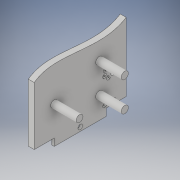
# Autodesk Inventor part: Case Right
Saved by Autodesk Inventor 2019 (Build 230136000, 136)
## iProperties
Created: 2022-04-25
Part Number: Case Right
Material: Generic
Document SubType Name: Modeling
Designer: Loxei
Density: 1 g/cm^3
Appearance: Default
Author: Loxei
Autodesk Inventor part; units mm, degrees
ref_plane "YZ Plane" through (0, 0, 0) normal (1, 0, 0) x (0, 1, 0)
ref_plane "XZ Plane" through (0, 0, 0) normal (0, 1, 0) x (-1, 0, 0)
ref_plane "XY Plane" through (0, 0, 0) normal (0, 0, 1) x (1, 0, 0)
sketch "Sketch1" plane through (0, 0, 0) normal (1, 0, 0) x (0, 1, 0)
  spline S0 degree 3 poles (-5.8666, 35) (13.8832, 21.2522) (-10.0462, -16.0043) (8.551, -35) knots 1 1 1 1 2 2 2 2
  line L0 (-5.8666, 35) -> (13.8832, 21.2522) construction
  line L1 (13.8832, 21.2522) -> (-10.0462, -16.0043) construction
  line L2 (-10.0462, -16.0043) -> (8.551, -35) construction
  line L3 (0, 65.172) -> (0, -65.172) construction
  line L4 (43.74, 0) -> (-43.74, 0) construction
  line L5 (-5.8666, 35) -> (-40.8666, 35)
  line L6 (-40.8666, 35) -> (-40.8666, 31)
  line L7 (-40.8666, 31) -> (-1.7165, 31)
  line L8 (-40.8666, 31) -> (-40.8666, -35)
  line L9 (-40.8666, -35) -> (8.551, -35)
  line L10 (-40.8666, -31) -> (5.392, -31)
  point P0 (0, 0)
  point P1 (0, 0)
  point P2 (-1.7165, 31)
  point P3 (0, 0)
  point P4 (0, 0)
  point P5 (0, 0)
  dimension "d0" = 35
  dimension "d1" = 4
  dimension "d2" = 4
  constraints: 16 end point, 4 midpoint, 3 perpendicular, 3 vertical, 2 horizontal, 2 parallel, 2 symmetric about line, 1 point on line, 6 other
  measures "d0" distance of L0.start L5.end
  measures "d1" distance of L5.end L6.end
  measures "d2" distance of L8.end L10.start
extrude "Extrusion1" add sketch "Sketch1" along normal blind 4 contours S0 L10 L8 L7
sketch "Sketch3" plane through (0, -40.8666, -31) normal (0, -1, 0) x (1, 0, 0)
  line L0 (2.3, 48.5) -> (4, 48.5)
  line L1 (4, 48.5) -> (4, 13.5)
  line L2 (4, 13.5) -> (2.3, 13.5)
  line L3 (2.3, 13.5) -> (2.3, 48.5)
  line L4 (0, 62) -> (0, 0) projected
  line L5 (0, 0) -> (4, 0) projected
  line L6 (4, 62) -> (4, 0) projected
  line L7 (0, 62) -> (4, 62) projected
  point P0 (0, 31)
  point P1 (4, 31)
  dimension "d5" = 1.7
  dimension "d6" = 35
  constraints: 8 end point, 2 midpoint, 2 parallel, 1 horizontal, 1 perpendicular
  measures "d5" distance of L1.end L2.end
  measures "d6" distance of L0.end L1.end
extrude "Extrusion2" add sketch "Sketch3" along normal blind 4.9 contours L0 L1 L2 L3
sketch "Sketch4" plane through (4, 0, 0) normal (1, 0, 0) x (0, 0, -1)
  circle A0 centre (12.8601, -10.8083) radius 2.425
  circle A1 centre (12.8601, -30.8083) radius 2.425
  line L0 (12.8601, -10.8083) -> (12.8601, -30.8083) construction
  circle A2 centre (-17.6399, -20.8083) radius 2.3037
  point P0 (0, 0)
  dimension "d11" = 4.85
  dimension "d12" = 4.85
  dimension "d13" = 20
  dimension "d14" = 4.6075
  dimension "d15" = 30.5
  constraints: 3 centre point, 2 end point, 1 vertical
  measures "d11" diameter of A0
  measures "d12" diameter of A1
  measures "d13" distance of L0.start L0.end
  measures "d14" diameter of A2
  measures "d15" distance from line of L0 A2.centre
extrude "Extrusion3" add sketch "Sketch4" along normal blind 17.2
chamfer "Chamfer1" distance 1.5 angle 45 1 edges at (2.3, -40.8666, 0)
sketch "Sketch5" plane through (4, 0, 0) normal (1, 0, 0) x (0, 0, -1)
  arc A0 (17.8302, -18.7899) -> (16.2318, -18.8201) centre (17.0282, -18.6552) ccw construction
  arc A1 (18.4232, -18.8896) -> (15.643, -18.942) centre (17.0282, -18.6552) ccw
  arc A2 (17.2372, -18.6903) -> (16.8207, -18.6981) centre (17.0282, -18.6552) ccw
  arc A3 (17.2372, -18.6903) -> (18.4232, -18.8896) centre (17.8302, -18.7899) ccw
  arc A4 (15.643, -18.942) -> (16.8207, -18.6981) centre (16.2318, -18.8201) ccw
  arc A5 (17.1142, -21.1556) -> (16.3411, -22.5549) centre (16.5965, -21.7828) ccw construction
  arc A6 (17.497, -20.6919) -> (16.1523, -23.1258) centre (16.5965, -21.7828) ccw
  arc A7 (16.7314, -21.6193) -> (16.5299, -21.984) centre (16.5965, -21.7828) ccw
  arc A8 (16.7314, -21.6193) -> (17.497, -20.6919) centre (17.1142, -21.1556) ccw
  arc A9 (16.1523, -23.1258) -> (16.5299, -21.984) centre (16.3411, -22.5549) ccw
  arc A10 (18.8049, -22.9585) -> (19.6302, -24.3277) centre (19.0892, -23.7205) ccw construction
  arc A11 (18.5947, -22.3952) -> (20.0302, -24.7766) centre (19.0892, -23.7205) ccw
  arc A12 (19.0151, -23.5219) -> (19.2302, -23.8787) centre (19.0892, -23.7205) ccw
  arc A13 (19.0151, -23.5219) -> (18.5947, -22.3952) centre (18.8049, -22.9585) ccw
  arc A14 (20.0302, -24.7766) -> (19.2302, -23.8787) centre (19.6302, -24.3277) ccw
  arc A15 (21.2117, -22.3958) -> (22.81, -22.3656) centre (22.0137, -22.5305) ccw construction
  arc A16 (20.6187, -22.2961) -> (23.3988, -22.2437) centre (22.0137, -22.5305) ccw
  arc A17 (21.8047, -22.4954) -> (22.2212, -22.4875) centre (22.0137, -22.5305) ccw
  arc A18 (21.8047, -22.4954) -> (20.6187, -22.2961) centre (21.2117, -22.3958) ccw
  arc A19 (23.3988, -22.2437) -> (22.2212, -22.4875) centre (22.81, -22.3656) ccw
  arc A20 (21.9277, -20.0301) -> (22.7007, -18.6308) centre (22.4454, -19.4029) ccw construction
  arc A21 (21.5449, -20.4938) -> (22.8895, -18.0599) centre (22.4454, -19.4029) ccw
  arc A22 (22.3105, -19.5663) -> (22.5119, -19.2017) centre (22.4454, -19.4029) ccw
  arc A23 (22.3105, -19.5663) -> (21.5449, -20.4938) centre (21.9277, -20.0301) ccw
  arc A24 (22.8895, -18.0599) -> (22.5119, -19.2017) centre (22.7007, -18.6308) ccw
  arc A25 (20.2369, -18.2272) -> (19.4116, -16.858) centre (19.9526, -17.4652) ccw construction
  arc A26 (20.4471, -18.7905) -> (19.0116, -16.4091) centre (19.9526, -17.4652) ccw
  arc A27 (20.0267, -17.6638) -> (19.8117, -17.307) centre (19.9526, -17.4652) ccw
  arc A28 (20.0267, -17.6638) -> (20.4471, -18.7905) centre (20.2369, -18.2272) ccw
  arc A29 (19.0116, -16.4091) -> (19.8117, -17.307) centre (19.4116, -16.858) ccw
  arc A30 (23.0405, -38.7872) -> (16.269, -38.8619) centre (19.6983, -42.7704) ccw construction
  arc A31 (23.7678, -37.9205) -> (15.5229, -38.0114) centre (19.6983, -42.7704) ccw
  arc A32 (22.3133, -39.6539) -> (17.0152, -39.7123) centre (19.6983, -42.7704) ccw
  arc A33 (22.3133, -39.6539) -> (23.7678, -37.9205) centre (23.0405, -38.7872) ccw
  arc A34 (15.5229, -38.0114) -> (17.0152, -39.7123) centre (16.269, -38.8619) ccw
  point P0 (0, 0)
  point P1 (19.5209, -20.5928)
  dimension "d30" = 360
  constraints: 70 point on circle, 35 centre point, 8 tangent, 73 other
extrude "Extrusion4" cut sketch "Sketch5" against normal blind 4
sketch "Sketch6" plane through (4, 0, 0) normal (1, 0, 0) x (0, 0, -1)
  line L0 (-17.5, -40.8666) -> (17.5, -40.8666) projected
  circle A0 centre (0, -43.1166) radius 1.575
  line L1 (17.5, -40.8666) -> (17.5, -45.7666) projected
  point P0 (0, 0)
  dimension "d32" = 3.15
  dimension "d33" = 2.25
  dimension "d36" = 17.5
  constraints: 1 centre point
  measures "d32" diameter of A0
  measures "d33" distance from line of L0 A0.centre
  measures "d36" distance from line of L1 A0.centre
extrude "Extrusion5" cut sketch "Sketch6" against normal blind 4
equation "\"d11\" = d12"
equation "\"d14\" = 0.95 * d12"
body "Solid1"
